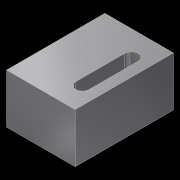
# Autodesk Inventor part: Part2
Saved by Autodesk Inventor 2021.1 (Build 251245000, 245)
## iProperties
Created: 2020-08-29
Part Number: Part2
Material: A5052
Document SubType Name: Modeling
Designer: Hashimoto
Mass: 3.56911 g
Surface Area: 9.47281 cm^2
Volume: 1.31681 cm^3
Density: 2.71043 g/cm^3
Appearance: アルミニウム - つや出し
Author: Hashimoto
Autodesk Inventor part; units mm, degrees
ref_plane "YZ Plane" through (0, 0, 0) normal (1, 0, 0) x (0, 1, 0)
ref_plane "XZ Plane" through (0, 0, 0) normal (0, 1, 0) x (-1, 0, 0)
ref_plane "XY Plane" through (0, 0, 0) normal (0, 0, 1) x (1, 0, 0)
sketch "スケッチ22" plane through (0, 0, 0) normal (0, 0, 1) x (1, 0, 0)
  line L0 (-6.9456, -9.9484) -> (6.9456, -9.9484)
  line L1 (6.9456, -9.9484) -> (6.9456, 9.9484)
  line L2 (6.9456, 9.9484) -> (-6.9456, 9.9484)
  line L3 (-6.9456, 9.9484) -> (-6.9456, -9.9484)
  line L4 (-6.9456, -9.9484) -> (6.9456, 9.9484) construction
  line L5 (6.9456, -9.9484) -> (-6.9456, 9.9484) construction
  point P0 (0, 0)
  constraints: 12 end point, 2 midpoint, 2 parallel, 1 horizontal, 1 perpendicular
extrude "押し出し14" add sketch "スケッチ22" along normal blind 5
sketch "スケッチ23" plane through (0, 0, 5) normal (0, 0, 1) x (1, 0, 0)
  line L0 (3.4613, 4.9054) -> (3.4613, -4.9971) construction
  line L1 (2.1075, 4.9054) -> (2.1075, -4.9971)
  line L2 (4.8151, -4.9971) -> (4.8151, 4.9054)
  arc A0 (4.8151, 4.9054) -> (2.1075, 4.9054) centre (3.4613, 4.9054) ccw
  arc A1 (2.1075, -4.9971) -> (4.8151, -4.9971) centre (3.4613, -4.9971) ccw
  point P0 (0, 0)
  point P1 (3.4613, -0.0458)
  constraints: 8 end point, 4 point on circle, 4 tangent, 2 centre point, 1 midpoint, 1 parallel, 1 vertical
extrude "押し出し15" cut sketch "スケッチ23" against normal blind 2
